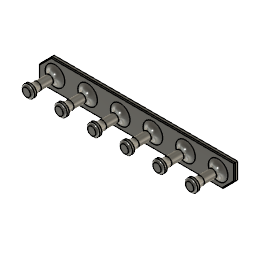
Thick Hanger (Autodesk Fusion 360 design; units mm, degrees)
part number: 2025-05-11-16-17-08-124
Autodesk Fusion 360 part; units mm, degrees
sketch "Sketch1" plane through (0, 0, 0) normal (0, 0, 1) x (1, 0, 0)
  line L0 (120, 20) -> (-120, 20)
  line L1 (-120, 20) -> (-120, -20)
  line L2 (-120, -20) -> (120, -20)
  line L3 (120, -20) -> (120, 20)
  line L4 (120, 20) -> (-120, -20) construction
  line L5 (-120, 20) -> (120, -20) construction
  dimension "d1" = 240
  dimension "d2" = 40
  dimension "d22" = 40
  dimension "d23" = 40
  dimension "d24" = 40
  dimension "d25" = 40
  dimension "d26" = 40
  dimension "d27" = 40
  dimension "d28" = 10
  dimension "d29" = 8.5
  dimension "d30" = 7.5
  dimension "d31" = 9
  dimension "d32" = 7.5
  dimension "d33" = 10.8
  constraint horizontal L0
  constraint perpendicular L0 L1
  constraint parallel L0 L2
  constraint parallel L1 L3
  constraint coincident L4 origin
  constraint coincident L5 origin
  measures "d1" distance of L1.end L2.end
  measures "d2" distance of L0.end L1.end
extrude "Extrude1" add sketch "Sketch1" along normal blind 5
sketch "Sketch2" plane through (0, 0, 5) normal (0, 0, 1) x (-1, 0, 0)
  line L0 (-120, 20) -> (-120, -20)
  line L1 (120, -20) -> (120, 20)
  line L2 (120, 20) -> (-120, 20)
  line L3 (120, -20) -> (-120, -20)
  line L4 (-120, -20) -> (-120, -16)
  line L5 (-120, -16) -> (120, -16)
  line L6 (120, -16) -> (120, -20)
  line L7 (-120, -20) -> (120, -20)
  dimension "d7" = 4
  constraint horizontal L3
  constraint vertical L4
  constraint horizontal L5
  constraint vertical L6
  constraint coincident L1.start L3.start
  measures "d7" distance of L1.start L5.end
extrude "Extrude3" add sketch "Sketch2" along normal blind 30 contours L0 L1 L3 L4 L5 L6 L7
sketch "Sketch3" plane through (0, 20, 0) normal (0, 1, 0) x (-1, 0, 0)
  line L0 (-120, 0) -> (120, 0)
  line L1 (120, 0) -> (120, 35)
  line L2 (120, 35) -> (-120, 35)
  line L3 (-120, 35) -> (-120, 0)
  line L4 (0, 35) -> (0, 0) construction
  line L5 (20.55, 35) -> (20.55, 0) construction
  line L6 (61.65, 35) -> (61.65, 0) construction
  line L7 (102.75, 35) -> (102.75, 0) construction
  line L8 (-20.55, 35) -> (-20.55, 0) construction
  line L9 (-61.65, 35) -> (-61.65, 0) construction
  line L10 (-102.75, 35) -> (-102.75, 0) construction
  line L11 (120, 17.5) -> (-120, 17.5) construction
  line L12 (27.95, 17.5) -> (24.25, 23.9086)
  line L13 (24.25, 23.9086) -> (16.85, 23.9086)
  line L14 (16.85, 23.9086) -> (13.15, 17.5)
  line L15 (13.15, 17.5) -> (16.85, 11.0914)
  line L16 (16.85, 11.0914) -> (24.25, 11.0914)
  line L17 (24.25, 11.0914) -> (27.95, 17.5)
  line L18 (-13.15, 17.5) -> (-16.85, 23.9086)
  line L19 (-16.85, 23.9086) -> (-24.25, 23.9086)
  line L20 (-24.25, 23.9086) -> (-27.95, 17.5)
  line L21 (-27.95, 17.5) -> (-24.25, 11.0914)
  line L22 (-24.25, 11.0914) -> (-16.85, 11.0914)
  line L23 (-16.85, 11.0914) -> (-13.15, 17.5)
  line L24 (-95.35, 17.5) -> (-99.05, 23.9086)
  line L25 (-99.05, 23.9086) -> (-106.45, 23.9086)
  line L26 (-106.45, 23.9086) -> (-110.15, 17.5)
  line L27 (-110.15, 17.5) -> (-106.45, 11.0914)
  line L28 (-106.45, 11.0914) -> (-99.05, 11.0914)
  line L29 (-99.05, 11.0914) -> (-95.35, 17.5)
  line L30 (95.35, 17.5) -> (99.05, 11.0914)
  line L31 (99.05, 11.0914) -> (106.45, 11.0914)
  line L32 (106.45, 11.0914) -> (110.15, 17.5)
  line L33 (110.15, 17.5) -> (106.45, 23.9086)
  line L34 (106.45, 23.9086) -> (99.05, 23.9086)
  line L35 (99.05, 23.9086) -> (95.35, 17.5)
  point P0 (20.55, 17.5)
  point P1 (-20.55, 17.5)
  point P2 (-102.75, 17.5)
  point P3 (102.75, 17.5)
  dimension "d10" = 20.55
  dimension "d11" = 41.1
  dimension "d12" = 41.1
  dimension "d13" = 41.1
  dimension "d14" = 41.1
  dimension "d15" = 20.55
  dimension "d16" = 7.4
  dimension "d17" = 7.4
  dimension "d18" = 7.4
  dimension "d19" = 7.4
  constraint midpoint L2 L4.start
  constraint coincident L4.end origin
  constraint coincident L2 L5.start
  constraint coincident L0 L5.end
  constraint perpendicular L0 L5
  constraint coincident L2 L6.start
  constraint coincident L0 L6.end
  constraint perpendicular L0 L6
  constraint coincident L0 L7.end
  constraint perpendicular L0 L7
  constraint coincident L2 L8.start
  constraint coincident L0 L8.end
  constraint perpendicular L0 L8
  constraint coincident L2 L9.start
  constraint coincident L0 L9.end
  constraint perpendicular L0 L9
  constraint coincident L2 L10.start
  constraint coincident L0 L10.end
  constraint perpendicular L0 L10
  constraint midpoint L1 L11.start
  constraint midpoint L3 L11.end
  constraint midpoint L5 P0
  constraint midpoint L8 P1
  constraint midpoint L10 P2
  constraint coincident L11 L30.start
  constraint midpoint L7 P3
  measures "d10" distance of L4 L5
  measures "d11" distance of L5 L6
  measures "d12" distance of L6 L7
  measures "d13" distance of L9 L10
  measures "d14" distance of L8 L9
  measures "d15" distance of L4 L8
  measures "d16" distance of L12.start P0
  measures "d17" distance of L18.start P1
  measures "d18" distance of L24.start P2
  measures "d19" distance of L30.start P3
extrude "Extrude4" add sketch "Sketch3" along normal blind 10 contours L12 L13 L14 L15 L16 L17 | L18 L19 L20 L21 L22 L23 | L24 L25 L26 L27 L28 L29 | L30 L31 L32 L33 L34 L35
extrude "Extrude8" cut 1 faces at (-40, -20, 1.6667) along direction (0, 1, 0) up to surface (36 mm away)
sketch "Sketch7" plane through (0, 16, 0) normal (0, -1, 0) x (1, 0, 0)
  line L0 (120, 0) -> (120, 35)
  line L1 (120, 35) -> (-120, 35)
  line L2 (-120, 35) -> (-120, 0)
  line L3 (-120, 0) -> (120, 0)
  line L4 (0, 35) -> (0, 0) construction
  line L5 (20, 35) -> (20, 0) construction
  line L6 (60, 35) -> (60, 0) construction
  line L7 (100, 35) -> (100, 0) construction
  line L8 (-20, 35) -> (-20, -2.1037) construction
  line L9 (-60, 35) -> (-60, 0) construction
  line L10 (-100, 35) -> (-100, 0) construction
  line L11 (120, 17.5) -> (-120, 17.5) construction
  circle A0 centre (-20, 16.4481) radius 5
  circle A1 centre (-60, 17.5) radius 5
  circle A2 centre (-100, 17.5) radius 5
  circle A3 centre (20, 17.5) radius 5
  circle A4 centre (60, 17.5) radius 5
  circle A5 centre (100, 17.5) radius 5
  dimension "d100" = 20
  dimension "d101" = 40
  dimension "d102" = 40
  dimension "d103" = 20
  dimension "d104" = 40
  dimension "d105" = 40
  dimension "d106" = 10
  dimension "d107" = 10
  dimension "d108" = 10
  dimension "d109" = 10
  dimension "d110" = 10
  dimension "d111" = 10
  constraint midpoint L1 L4.start
  constraint coincident L4.end origin
  constraint coincident L1 L5.start
  constraint coincident L3 L5.end
  constraint perpendicular L3 L5
  constraint coincident L1 L6.start
  constraint coincident L3 L6.end
  constraint perpendicular L3 L6
  constraint coincident L1 L7.start
  constraint coincident L3 L7.end
  constraint perpendicular L3 L7
  constraint coincident L1 L8.start
  constraint perpendicular L3 L8
  constraint coincident L1 L9.start
  constraint coincident L3 L9.end
  constraint perpendicular L3 L9
  constraint coincident L1 L10.start
  constraint coincident L3 L10.end
  constraint perpendicular L3 L10
  constraint midpoint L0 L11.start
  constraint midpoint L2 L11.end
  constraint midpoint L8 A0.centre
  constraint midpoint L9 A1.centre
  constraint midpoint L10 A2.centre
  constraint midpoint L5 A3.centre
  constraint midpoint L6 A4.centre
  constraint midpoint L7 A5.centre
  measures "d100" distance of L4 L5
  measures "d101" distance of L5 L6
  measures "d102" distance of L6 L7
  measures "d103" distance of L4 L8
  measures "d104" distance of L8 L9
  measures "d105" distance of L9 L10
  measures "d106" diameter of A0
  measures "d107" diameter of A1
  measures "d108" diameter of A2
  measures "d109" diameter of A3
  measures "d110" diameter of A4
  measures "d111" diameter of A5
extrude "Extrude9" add sketch "Sketch7" along normal blind 30 contours A0 | A1 | A2 | A3 | A4 | A5
sketch "Sketch8" plane through (0, -14, 0) normal (0, -1, 0) x (1, 0, 0)
  circle A0 centre (-100, 17.5) radius 5
  circle A1 centre (-100, 17.5) radius 7.5
  dimension "d114" = 15
  constraint concentric A0 A1
  measures "d114" diameter of A1
extrude "Extrude10" add sketch "Sketch8" along normal blind 5 contours A0 | A1
sketch "Sketch9" plane through (0, -14, 0) normal (0, -1, 0) x (1, 0, 0)
  circle A0 centre (-60, 17.5) radius 5
  circle A1 centre (-60, 17.5) radius 7.5
  dimension "d117" = 15
  constraint concentric A0 A1
  measures "d117" diameter of A1
extrude "Extrude11" add sketch "Sketch9" along normal blind 5 contours A0 | A1
sketch "Sketch10" plane through (0, -14, 0) normal (0, -1, 0) x (1, 0, 0)
  circle A0 centre (-20, 16.4481) radius 5
  circle A1 centre (-20, 16.4481) radius 7.5
  dimension "d120" = 15
  constraint concentric A0 A1
  measures "d120" diameter of A1
extrude "Extrude12" add sketch "Sketch10" along normal blind 5 contours A0 | A1
sketch "Sketch11" plane through (0, -14, 0) normal (0, -1, 0) x (1, 0, 0)
  circle A0 centre (20, 17.5) radius 5
  circle A1 centre (20, 17.5) radius 7.5
  dimension "d123" = 15
  constraint concentric A0 A1
  measures "d123" diameter of A1
extrude "Extrude13" add sketch "Sketch11" along normal blind 5 contours A0 | A1
sketch "Sketch12" plane through (0, -14, 0) normal (0, -1, 0) x (1, 0, 0)
  circle A0 centre (60, 17.5) radius 5
  circle A1 centre (60, 17.5) radius 7.5
  dimension "d126" = 15
  constraint concentric A0 A1
  measures "d126" diameter of A1
extrude "Extrude14" add sketch "Sketch12" along normal blind 5 contours A0 | A1
sketch "Sketch13" plane through (0, -14, 0) normal (0, -1, 0) x (1, 0, 0)
  circle A0 centre (100, 17.5) radius 5
  circle A1 centre (100, 17.5) radius 7.5
  dimension "d129" = 15
  constraint concentric A0 A1
  measures "d129" diameter of A1
extrude "Extrude15" add sketch "Sketch13" along normal blind 5 contours A0 | A1
fillet "Fillet3" radius 15 6 edges at (95.3384, -14, 15.6919) (55.3384, -14, 15.6919) (15.3384, -14, 15.6919) (-24.6616, -14, 14.6401) (-64.6616, -14, 15.6919) (-104.6616, -14, 15.6919)
fillet "Fillet4" radius 2.5 6 edges at (93.0075, -19, 14.7879) (53.0075, -19, 14.7879) (13.0075, -19, 14.7879) (-26.9925, -19, 13.736) (-66.9925, -19, 14.7879) (-106.9925, -19, 14.7879)
chamfer "Chamfer15" distance 15 angle 45 2 edges at (-120, 18, 35) (120, 18, 0)
chamfer "Chamfer16" distance 2 angle 45 24 edges at (102.75, 30, 23.9086) (108.3, 30, 20.7043) (108.3, 30, 14.2957) (102.75, 30, 11.0914) (97.2, 30, 14.2957) (97.2, 30, 20.7043) (20.55, 30, 23.9086) (26.1, 30, 20.7043) (26.1, 30, 14.2957) (20.55, 30, 11.0914) (15, 30, 14.2957) (15, 30, 20.7043) (-20.55, 30, 23.9086) (-15, 30, 20.7043) (-15, 30, 14.2957) (-20.55, 30, 11.0914) (-26.1, 30, 14.2957) (-26.1, 30, 20.7043) (-102.75, 30, 23.9086) (-97.2, 30, 20.7043) (-97.2, 30, 14.2957) (-102.75, 30, 11.0914) (-108.3, 30, 14.2957) (-108.3, 30, 20.7043)
chamfer "Chamfer17" distance 1 angle 45 6 edges at (7.5, 16, 35) (-112.5, 16, 27.5) (-120, 16, 10) (-7.5, 16, 0) (120, 16, 25) (112.5, 16, 7.5)
fillet "Fillet5" radius 7 6 edges at (-104.6616, 16, 19.3081) (-64.6616, 16, 19.3081) (-24.6616, 16, 18.2562) (15.3384, 16, 19.3081) (55.3384, 16, 19.3081) (95.3384, 16, 19.3081)
fillet "Fillet6" radius 1.5 24 edges at (99.05, 24, 23.9086) (106.45, 24, 23.9086) (110.15, 24, 17.5) (106.45, 24, 11.0914) (16.85, 24, 23.9086) (24.25, 24, 23.9086) (27.95, 24, 17.5) (24.25, 24, 11.0914) (-24.25, 24, 23.9086) (-16.85, 24, 23.9086) (-13.15, 24, 17.5) (-16.85, 24, 11.0914) (-106.45, 24, 23.9086) (-99.05, 24, 23.9086) (-95.35, 24, 17.5) (-99.05, 24, 11.0914) (95.35, 24, 17.5) (99.05, 24, 11.0914) (13.15, 24, 17.5) (16.85, 24, 11.0914) (-27.95, 24, 17.5) (-24.25, 24, 11.0914) (-110.15, 24, 17.5) (-106.45, 24, 11.0914)
equation "d22 = ( 240 / 6 ) * 1 mm"
equation "d60 = ( 80.8 / 3 ) * 1 mm"
equation "d61 = ( 80.8 / 3 ) * 1 mm"
equation "d64 = ( 26.933 / 2 ) * 1 mm"
equation "d65 = ( 26.933 / 2 ) * 1 mm"
equation "d73 = ( 80.8 / 3 ) * 1 mm"
equation "d74 = ( 80.8 / 3 ) * 1 mm"
equation "d77 = ( 26.933 / 2 ) * 1 mm"
equation "d81 = ( 17.5 / 2 ) * 1 mm"
